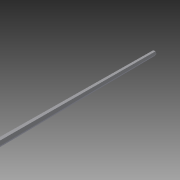
# Autodesk Inventor part: bigShaft2
Saved by Autodesk Inventor 2015 (Build 190159000, 159)
## iProperties
Created: 2016-04-21
Part Number: bigShaft2
Material: Generic
Document SubType Name: Modeling
Designer: Administrator
Density: 1 g/cm^3
Appearance: Default
Author: Administrator
Autodesk Inventor part; units mm, degrees
ref_plane "YZ Plane" through (0, 0, 0) normal (1, 0, 0) x (0, 1, 0)
ref_plane "XZ Plane" through (0, 0, 0) normal (0, 1, 0) x (-1, 0, 0)
ref_plane "XY Plane" through (0, 0, 0) normal (0, 0, 1) x (1, 0, 0)
sketch "Sketch1" plane through (0, 0, 0) normal (0, 0, 1) x (1, 0, 0)
  line L0 (2.6781, 6.36) -> (10.0219, 6.36) projected
  line L1 (-0.9939, 0) -> (2.6781, 6.36) projected
  line L2 (2.6781, -6.36) -> (-0.9939, 0) projected
  line L3 (10.0219, -6.36) -> (2.6781, -6.36) projected
  line L4 (13.6939, 0) -> (10.0219, -6.36) projected
  line L5 (10.0219, 6.36) -> (13.6939, 0) projected
  point P0 (0, 0)
extrude "Extrusion1" add sketch "Sketch1" along normal blind 457.2
body "Solid1"
